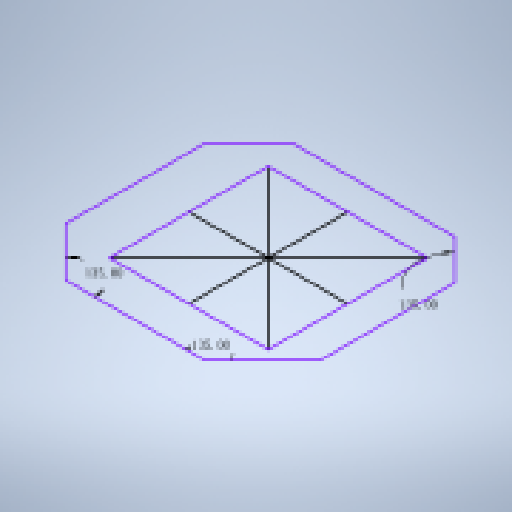
# Autodesk Inventor part: 底板
Saved by Autodesk Inventor 2025.2 (Build 292293000, 293)
## iProperties
Created: 2025-10-21
Part Number: 底板
Material: 常规
Document SubType Name: Modeling
Designer: BO‘S_SLAVE
Density: 1 g/cm^3
Appearance: 默认
Author: BO‘S_SLAVE
Autodesk Inventor part; units mm, degrees
ref_plane "YZ Plane" through (0, 0, 0) normal (1, 0, 0) x (0, 1, 0)
ref_plane "XZ Plane" through (0, 0, 0) normal (0, 1, 0) x (-1, 0, 0)
ref_plane "XY Plane" through (0, 0, 0) normal (0, 0, 1) x (1, 0, 0)
sketch "草图4" plane through (0, 0, 0) normal (0, 1, 0) x (-1, 0, 0)
  line L0 (-21.2132, 21.2132) -> (21.2132, 21.2132)
  line L1 (21.2132, 21.2132) -> (21.2132, -21.2132)
  line L2 (21.2132, -21.2132) -> (-21.2132, -21.2132)
  line L3 (-21.2132, -21.2132) -> (-21.2132, 21.2132)
  line L4 (0, 21.2132) -> (0, -21.2132)
  line L5 (-21.2132, 0) -> (21.2132, 0)
  line L6 (-21.2132, 21.2132) -> (21.2132, -21.2132)
  line L7 (21.2132, 21.2132) -> (-21.2132, -21.2132)
  line L8 (-12.4264, -30) -> (-30, -12.4264)
  line L9 (-30, -12.4264) -> (-30, 12.4264)
  line L10 (-30, 12.4264) -> (-12.4264, 30)
  line L11 (-12.4264, 30) -> (12.4264, 30)
  line L12 (12.4264, 30) -> (30, 12.4264)
  line L13 (30, 12.4264) -> (30, -12.4264)
  line L14 (30, -12.4264) -> (12.4264, -30)
  line L15 (12.4264, -30) -> (-12.4264, -30)
  line L16 (-16.5685, -40) -> (-40, -16.5685)
  line L17 (-40, -16.5685) -> (-40, 16.5685)
  line L18 (-40, 16.5685) -> (-16.5685, 40)
  line L19 (-16.5685, 40) -> (16.5685, 40)
  line L20 (16.5685, 40) -> (40, 16.5685)
  line L21 (40, 16.5685) -> (40, -16.5685)
  line L22 (40, -16.5685) -> (16.5685, -40)
  line L23 (16.5685, -40) -> (-16.5685, -40)
  point P0 (0, 0)
  point P1 (0, 0)
  point P2 (0, 0)
  point P3 (0, 0)
  dimension "d261" = 60
  dimension "d268" = 10
  constraints: 48 end point, 6 midpoint, 3 coincident, 3 parallel, 2 perpendicular, 1 horizontal, 34 other
  measures "d261" distance of L0.end L2.end
  measures "d268" distance between parallel lines of L15 L23
extrude "拉伸5" add sketch "草图4" along normal blind 3 contours L10 L11 L12 L0 | L6 L5 L3 | L0 L4 L6 | L3 L8 L9 L10 | L0 L7 L4 | L5 L7 L3 | L6 L2 L4 | L7 L1 L5 | L5 L1 L6 | L4 L2 L7 | L12 L13 L14 L1 | L2 L14 L15 L8 | L16 L17 L18 L19 L20 L21 L22 L23
